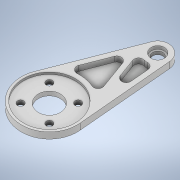
# Autodesk Inventor part: 足首_独立ピッチ_1_1
Saved by Autodesk Inventor 2020.4 (Build 244396000, 396)
## iProperties
Created: 2021-09-01
Part Number: 足首_独立ピッチ_1_1
Material: アルミニウム 2014-T4
Document SubType Name: Modeling
Designer: naoki
Density: 2.8 g/cm^3
Appearance: 滑らか - 淡い灰色
Author: naoki
Autodesk Inventor part; units mm, degrees
ref_plane "YZ Plane" through (0, 0, 0) normal (1, 0, 0) x (0, 1, 0)
ref_plane "XZ Plane" through (0, 0, 0) normal (0, 1, 0) x (-1, 0, 0)
ref_plane "XY Plane" through (0, 0, 0) normal (0, 0, 1) x (1, 0, 0)
derived "下半身全体像_1_1.ipt"
sketch "スケッチ1" plane through (0, 0, 0) normal (0, 0, 1) x (1, 0, 0)
  circle A0 centre (0, 0) radius 10.5 construction
  line L0 (0, 0) -> (-12, 0) construction
  arc A1 (0, 16) -> (-12, 10.583) centre (0, 0) ccw construction
  arc A2 (-12, -10.583) -> (0, -16) centre (0, 0) ccw construction
  line L1 (0, 16) -> (39.5, 16) construction
  line L2 (39.5, 16) -> (39.5, -16) construction
  line L3 (39.5, -16) -> (0, -16) construction
  circle A3 centre (1, 13.5) radius 1.35 projected
  circle A4 centre (1, -13.5) radius 1.35 projected
  circle A5 centre (28, 13.5) radius 1.35 projected
  circle A6 centre (28, -13.5) radius 1.35 projected
  line L4 (1, 13.5) -> (1, -13.5) construction
  line L5 (1, -13.5) -> (28, -13.5) construction
  line L6 (1, 13.5) -> (28, 13.5) construction
  line L7 (28, 13.5) -> (28, -13.5) construction
  line L8 (0, 0) -> (1, 0) construction
  line L9 (32, 120) -> (32, 20) construction
  line L10 (0, 0) -> (0, 0) construction
  circle A7 centre (32, 120) radius 4.05 projected
  line L11 (0, 140) -> (0, 40) construction
  circle A8 centre (0, 40) radius 4.05 projected
  line L12 (0, 0) -> (0, -100) construction
  line L13 (32, 20) -> (32, -80) construction
  line L14 (0, 0) -> (0, 40) construction
  circle A9 centre (32, 20) radius 6.5 construction
  line L15 (32, 23.5218) -> (35.05, 21.7609) construction
  line L16 (35.05, 21.7609) -> (35.05, 18.2391) construction
  line L17 (35.05, 18.2391) -> (32, 16.4782) construction
  line L18 (32, 16.4782) -> (28.95, 18.2391) construction
  line L19 (28.95, 18.2391) -> (28.95, 21.7609) construction
  line L20 (28.95, 21.7609) -> (32, 23.5218) construction
  line L21 (21.5, 152) -> (61, 152) construction
  line L22 (61, 152) -> (61, 100.5) construction
  line L23 (61, 100.5) -> (21.5, 100.5) construction
  line L24 (21.5, 100.5) -> (21.5, 152) construction
  line L25 (21.5, 140) -> (61, 140) construction
  line L26 (16, 150.5) -> (66.5, 150.5) construction
  line L27 (66.5, 150.5) -> (66.5, 129.5) construction
  line L28 (66.5, 129.5) -> (16, 129.5) construction
  line L29 (16, 129.5) -> (16, 150.5) construction
  circle A10 centre (0, 140) radius 10.5 construction
  line L30 (-13.5, 139) -> (13.5, 139) construction
  line L31 (13.5, 139) -> (13.5, 112) construction
  line L32 (13.5, 112) -> (-13.5, 112) construction
  line L33 (-13.5, 112) -> (-13.5, 139) construction
  circle A11 centre (-13.5, 139) radius 1.35 projected
  circle A12 centre (13.5, 139) radius 1.35 projected
  circle A13 centre (-13.5, 112) radius 1.35 projected
  circle A14 centre (13.5, 112) radius 1.35 projected
  line L34 (-12, 10.583) -> (-12, -10.583) construction
  circle A15 centre (0, -100) radius 4.05 construction
  circle A16 centre (32, -80) radius 4.05 construction
  circle A17 centre (0, -100) radius 10.5 construction
  line L35 (32, -80) -> (0, -100) construction
  line L36 (45, -60.5) -> (77.5, -60.5) construction
  line L37 (77.5, -60.5) -> (77.5, -112) construction
  line L38 (77.5, -112) -> (45, -112) construction
  line L39 (45, -112) -> (45, -60.5) construction
  line L40 (45, -100) -> (77.5, -100) construction
  line L41 (39.5, -89.5) -> (83, -89.5) construction
  line L42 (83, -89.5) -> (83, -110.5) construction
  line L43 (83, -110.5) -> (39.5, -110.5) construction
  line L44 (39.5, -110.5) -> (39.5, -89.5) construction
  line L45 (1, -86.5) -> (28, -86.5) construction
  line L46 (28, -86.5) -> (28, -113.5) construction
  line L47 (28, -113.5) -> (1, -113.5) construction
  line L48 (1, -113.5) -> (1, -86.5) construction
  circle A18 centre (1, -86.5) radius 1.35 projected
  circle A19 centre (1, -113.5) radius 1.35 projected
  circle A20 centre (28, -113.5) radius 1.35 projected
  circle A21 centre (28, -86.5) radius 1.35 projected
  circle A22 centre (32, 20) radius 4.05 projected
  circle A23 centre (32, 20) radius 4.05 projected
  line L49 (10.583, 152) -> (-10.583, 152) construction
  line L50 (16, 140) -> (16, 100.5) construction
  line L51 (16, 100.5) -> (-16, 100.5) construction
  line L52 (-16, 100.5) -> (-16, 140) construction
  arc A24 (16, 140) -> (10.583, 152) centre (0, 140) ccw construction
  arc A25 (-10.583, 152) -> (-16, 140) centre (0, 140) ccw construction
  line L53 (-12, -89.417) -> (-12, -110.583) construction
  line L54 (0, -84) -> (39.5, -84) construction
  line L55 (39.5, -84) -> (39.5, -116) construction
  line L56 (39.5, -116) -> (0, -116) construction
  arc A26 (0, -84) -> (-12, -89.417) centre (0, -100) ccw construction
  arc A27 (-12, -110.583) -> (0, -116) centre (0, -100) ccw construction
  circle A28 centre (-8.5, 0) radius 1.35 projected
  circle A29 centre (0, 0) radius 8.5 construction
  line L57 (35.05, 121.7609) -> (35.05, 118.2391) construction
  line L58 (35.05, 118.2391) -> (32, 116.4782) construction
  line L59 (32, 116.4782) -> (28.95, 118.2391) construction
  line L60 (28.95, 118.2391) -> (28.95, 121.7609) construction
  line L61 (28.95, 121.7609) -> (32, 123.5218) construction
  line L62 (32, 123.5218) -> (35.05, 121.7609) construction
  line L63 (0, 152) -> (0, 140) construction
  line L64 (0, 140) -> (0, 139) construction
  circle A30 centre (0, -100) radius 5.05
  circle A31 centre (0, -100) radius 12 construction
  circle A32 centre (0, -100) radius 11 construction
  circle A33 centre (0, -100) radius 13
  circle A34 centre (-8.5, -100) radius 1.35
  line L65 (-24.9932, -100) -> (93.0564, -100) construction
  circle A35 centre (0, -108.5) radius 1.35
  circle A36 centre (8.5, -100) radius 1.35
  circle A37 centre (0, -91.5) radius 1.35
  circle A38 centre (32, -80) radius 2.25
  arc A39 (27.76, -82.65) -> (31.2277, -84.94) centre (32, -80) ccw
  line L66 (30.3091, -75.2946) -> (-4.3963, -87.7659)
  line L67 (35.4886, -83.5818) -> (9.0705, -109.3127)
  arc A40 (30.3091, -75.2946) -> (27.2211, -78.5295) centre (32, -80) ccw construction
  arc A41 (35.4886, -83.5818) -> (30.3091, -75.2946) centre (32, -80) ccw
  circle A42 centre (-8.5, -100) radius 2.5 construction
  circle A43 centre (0, -100) radius 12.01
  line L68 (31.2277, -84.94) -> (13.8905, -101.8262)
  line L69 (27.2211, -78.5295) -> (4.4453, -86.7139)
  arc A44 (13.8905, -101.8262) -> (4.4453, -86.7139) centre (0, -100) ccw
  arc A45 (27.2211, -78.5295) -> (27.76, -82.65) centre (32, -80) ccw
  arc A46 (31.2277, -84.94) -> (35.4886, -83.5818) centre (32, -80) ccw construction
  line L70 (13.8905, -101.8262) -> (27.2211, -78.5295)
  line L71 (13.8477, -97.8739) -> (24.3204, -79.5718)
  circle A47 centre (32, -80) radius 3.01
  point P0 (66.5, 140)
  point P1 (39.5, 0)
  point P2 (83, -100)
  point P3 (1, -100)
  point P4 (-12, -100)
  point P5 (39.5, -100)
  point P6 (83, -100)
  dimension "d5" = 17
  dimension "d2" = 10.1
  dimension "d3" = 1
  dimension "d4" = 1
  dimension "d14" = 2.7
  dimension "d15" = 8.5
  dimension "d18" = 360
  dimension "d20" = 4.5
  dimension "d21" = 10
  dimension "d22" = 5
  dimension "d23" = 0.01
  dimension "d25" = 2
  dimension "d26" = 2
  dimension "d27" = 2
  dimension "d29" = 2
  dimension "d37" = 6.02
  constraints: 18 centre point, 15 point on circle, 14 end point, 10 coincident, 8 tangent, 4 point on line, 3 parallel, 2 horizontal, 1 horizontal alignment, 1 midpoint, 1 perpendicular, 1 vertical, 11 other
  measures "d2" diameter of A30
  measures "d3" radial gap between concentric circles of A32 A31
  measures "d4" radial gap between concentric circles of A33 A31
  measures "d14" diameter of A34
  measures "d15" distance of A34.centre A15.centre
  measures "d20" diameter of A38
  measures "d21" diameter of A39
  measures "d22" diameter of A42
  measures "d23" radial gap between concentric circles of A43 A31
  measures "d25" distance between parallel lines of L66 L69
  measures "d26" distance between parallel lines of L67 L68
  measures "d27" radial gap between concentric circles of A44 A43
  measures "d29" distance between parallel lines of L71 L70
  measures "d37" diameter of A47
extrude "押し出し1" add sketch "スケッチ1" along normal blind 3 contours A18 A33 L66 | A18 L66 A41 L67 A33 | A33 A19 A18 | A18 A33 | A18 A33 L66 | A19 A33 | L68 A21 | A44 L71 L69 L70 picked at (0.8848, -112.6976) picked at (28.7147, -87.4511)
extrude "押し出し2" add sketch "スケッチ1" along normal blind 0.5 contours A21 L68 | A21 L68 L70 A45 A39 | A44 L69 L71 picked at (27.8851, -87.13)
extrude "押し出し3" add sketch "スケッチ1" along normal blind 2 contours A43
fillet "フィレット1" radius 2 6 edges at (24.3204, -79.5718, 1.75) (27.2211, -78.5295, 1.75) (4.4453, -86.7139, 1.75) (13.8477, -97.8739, 1.75) (13.8905, -101.8262, 1.75) (31.2277, -84.94, 1.75)
extrude "押し出し4" add sketch "スケッチ1" along normal blind 1.5 contours A47
equation "\"d15\" = 0.5 * d5"
equation "\"d26\" = d25"
equation "\"d27\" = d25"
